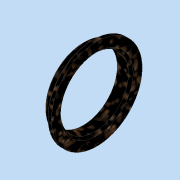
# Autodesk Inventor part: Gleit überlast
Saved by Autodesk Inventor 2021 (Build 250183000, 183)
## iProperties
Created: 2024-03-14
Part Number: Gleit überlast
Material: Generic
Document SubType Name: Modeling
Designer: Nokia
Density: 1 g/cm^3
Appearance: Dirt - Dark Brown
Author: Nokia
Autodesk Inventor part; units mm, degrees
ref_plane "YZ Plane" through (0, 0, 0) normal (1, 0, 0) x (0, 1, 0)
ref_plane "XZ Plane" through (0, 0, 0) normal (0, 1, 0) x (-1, 0, 0)
ref_plane "XY Plane" through (0, 0, 0) normal (0, 0, 1) x (1, 0, 0)
sketch "Sketch1" plane through (0, 0, 0) normal (0, 0, 1) x (1, 0, 0)
  line L0 (0, 0) -> (0, 15)
  line L1 (0, 15) -> (-6, 15)
  line L2 (-6, 15) -> (-6, 17)
  line L3 (-6, 17) -> (-2, 17)
  line L4 (-2, 17) -> (-2, 20)
  line L5 (-2, 20) -> (0, 20)
  line L6 (0, 20) -> (0, 15)
  line L7 (3.3032, 0) -> (-10.2133, 0)
  dimension "d0" = 15
  dimension "d1" = 6
  dimension "d2" = 2
  dimension "d3" = 4
  dimension "d4" = 3
  constraints: 16 end point, 6 perpendicular, 1 horizontal, 1 point on line, 1 vertical
  measures "d0" distance of L0.start L0.end
  measures "d1" distance of L0.end L1.end
  measures "d2" distance of L1.end L2.end
  measures "d3" distance of L2.end L3.end
  measures "d4" distance of L3.end L4.end
revolve "Revolution1" add sketch "Sketch1" angle 360 about axis through (3.3032, 0, 0) along (-1, 0, 0)
chamfer "Chamfer1" distance 1 angle 45 1 edges at (0, -15, 0)
chamfer "Chamfer2" distance 0.5 angle 45 2 edges at (-2, -20, 0) (-6, -17, 0)
body "Solid1"
